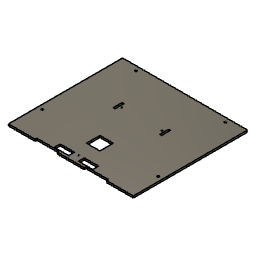
tablet_back_plate (Autodesk Fusion 360 design; units mm, degrees)
Autodesk Fusion 360 part; units mm, degrees
note: some values were not read from the file. Set by a fixed rule: the direction of a hole.
sketch "スケッチ1" plane through (0, 0, 0) normal (0, 1, 0) x (1, 0, 0)
  line L0 (140, 0) -> (140, 256)
  line L1 (140, 256) -> (-140, 256)
  line L2 (-140, 256) -> (-140, 0)
  line L3 (-54, 169) -> (-50, 169)
  line L4 (-50, 169) -> (-50, 149)
  line L5 (-50, 149) -> (-54, 149)
  line L6 (-54, 149) -> (-54, 169)
  line L7 (50, 169) -> (54, 169)
  line L8 (54, 169) -> (54, 149)
  line L9 (54, 149) -> (50, 149)
  line L10 (50, 149) -> (50, 169)
  line L11 (-50, 159) -> (-45, 159)
  line L12 (50, 159) -> (45, 159)
  line L13 (-130, 66) -> (-130, 246)
  line L14 (-130, 246) -> (130, 246)
  line L15 (130, 246) -> (130, 66)
  line L16 (-140, 0) -> (-80, 0)
  line L17 (-80, 0) -> (-80, 4)
  line L18 (-80, 4) -> (-30, 4)
  line L19 (-30, 4) -> (-30, 0)
  line L20 (-30, 0) -> (30, 0)
  line L21 (30, 0) -> (30, 4)
  line L22 (30, 4) -> (80, 4)
  line L23 (80, 4) -> (80, 0)
  line L24 (80, 0) -> (140, 0)
  line L25 (0, 0) -> (0, 17.5)
  line L26 (15, 80) -> (-15, 80)
  line L27 (-15, 80) -> (-15, 50)
  line L28 (-15, 50) -> (15, 50)
  line L29 (15, 50) -> (15, 80)
  line L30 (15, 80) -> (-15, 50) construction
  line L31 (-15, 80) -> (15, 50) construction
  point P0 (-100, 246)
  point P1 (100, 246)
  point P2 (0, 65)
  dimension "d1" = 256
  dimension "d4" = 50
  dimension "d6" = 20
  dimension "d7" = 4
  dimension "d8" = 5
  dimension "d14" = 10
  dimension "d15" = 10
  dimension "d16" = 10
  dimension "d17" = 180
  dimension "d18" = 100
  dimension "d19" = 100
  dimension "d25" = 60
  dimension "d26" = 60
  dimension "d27" = 60
  dimension "d28" = 140
  dimension "d29" = 140
  dimension "d30" = 4
  dimension "d32" = 13.5
  dimension "d33" = 50
  dimension "d34" = 30
  dimension "d35" = 30
  dimension "d41" = 50
  dimension "d42" = 149
  constraint vertical L0
  constraint horizontal L1
  constraint vertical L2
  constraint horizontal L3
  constraint vertical L4
  constraint horizontal L5
  constraint vertical L6
  constraint horizontal L7
  constraint vertical L8
  constraint horizontal L9
  constraint vertical L10
  constraint midpoint L4 L11.start
  constraint perpendicular L4 L11
  constraint midpoint L10 L12.start
  constraint perpendicular L10 L12
  constraint equal L3 L7
  constraint collinear L3 L7
  constraint collinear L5 L9
  constraint equal L11 L12
  constraint vertical L13
  constraint perpendicular L13 L14
  constraint perpendicular L14 L15
  constraint equal L13 L15
  constraint coincident L14 P0
  constraint coincident L14 P1
  constraint perpendicular L2 L16
  constraint perpendicular L16 L17
  constraint perpendicular L17 L18
  constraint perpendicular L16 L19
  constraint perpendicular L19 L20
  constraint perpendicular L20 L21
  constraint perpendicular L19 L22
  constraint perpendicular L22 L23
  constraint perpendicular L23 L24
  constraint coincident L0.start L24
  constraint coincident L0.start L24.end
  constraint collinear L16 L20
  constraint collinear L20 L24
  constraint midpoint L25.start L20
  constraint collinear L18 L22
  constraint coincident L25.start origin
  constraint perpendicular L20 L25
  constraint horizontal L26
  constraint perpendicular L26 L27
  constraint parallel L26 L28
  constraint parallel L27 L29
  constraint coincident L30 P2
  constraint coincident L31 P2
  constraint vertical L25.start P2
  measures "d1" distance of L0.start L0.end
  measures "d4" distance of L25.start L4
  measures "d6" distance of L7.end L8.end
  measures "d7" distance of L8.end L9.end
  measures "d8" distance of L12.start L12.end
  measures "d14" distance of L1 L14
  measures "d15" distance of L2 L13
  measures "d16" distance of L0 L15
  measures "d17" distance of L13.start L13.end
  measures "d18" horizontal distance of L25.start P0
  measures "d19" horizontal distance of L25.start P1
  measures "d25" distance of L19.end L20.end
  measures "d26" distance of L2.end L16.end
  measures "d27" distance of L23.end L0.start
  measures "d28" distance of L25.start L2
  measures "d29" distance of L25.start L0
  measures "d30" distance of L18 L20
  measures "d32" distance of L18 L25.end
  measures "d33" distance of L20 L28
  measures "d34" distance of L26.end L27.end
  measures "d35" distance of L26.start L26.end
  measures "d41" distance of L25.start L10
  measures "d42" distance of L25.start L9
extrude "押し出し1" add sketch "スケッチ1" along normal blind 4
hole "穴1" at (-45, 0, -159) at (45, 0, -159) at (0, 0, -17.5) direction (0, 1, 0) diameter 3.2 depth 4 tip angle 118
hole "穴2" at (100, 0, -246) at (130, 0, -66) at (-130, 0, -66) at (-100, 0, -246) direction (0, 1, 0) diameter 4.3 end through all
fillet "フィレット1" radius 1 2 edges at (140, 2, -256) (-140, 2, -256)
sketch "スケッチ2" plane through (0, 4, 0) normal (0, 1, 0) x (-1, 0, 0)
  arc A0 (139, -256) -> (140, -255) centre (139, -255) ccw
  line L0 (140, -255) -> (140, 0)
  line L1 (140, 0) -> (80, 0)
  line L2 (80, 0) -> (80, -4)
  line L3 (80, -4) -> (30, -4)
  line L4 (30, -4) -> (30, 0)
  line L5 (30, 0) -> (-30, 0)
  line L6 (-30, 0) -> (-30, -4)
  line L7 (-30, -4) -> (-80, -4)
  line L8 (-80, -4) -> (-80, 0)
  line L9 (-80, 0) -> (-140, 0)
  line L10 (-140, 0) -> (-140, -255)
  arc A1 (-140, -255) -> (-139, -256) centre (-139, -255) ccw
  line L11 (-139, -256) -> (139, -256)
  circle A2 centre (130, -66) radius 2.15
  circle A3 centre (-100, -246) radius 2.15
  circle A4 centre (-130, -66) radius 2.15
  circle A5 centre (100, -246) radius 2.15
  circle A6 centre (-45, -159) radius 1.6
  circle A7 centre (45, -159) radius 1.6
  circle A8 centre (0, -17.5) radius 1.6
  line L12 (-54, -149) -> (-50, -149)
  line L13 (-50, -149) -> (-50, -169)
  line L14 (-50, -169) -> (-54, -169)
  line L15 (-54, -169) -> (-54, -149)
  line L16 (-15, -80) -> (-15, -50)
  line L17 (-15, -50) -> (15, -50)
  line L18 (15, -50) -> (15, -80)
  line L19 (15, -80) -> (-15, -80)
  line L20 (50, -149) -> (54, -149)
  line L21 (54, -149) -> (54, -169)
  line L22 (54, -169) -> (50, -169)
  line L23 (50, -169) -> (50, -149)
  line L24 (-43, -6) -> (-11, -6)
  line L25 (-11, -6) -> (-11, -19)
  line L26 (-11, -19) -> (-43, -19)
  line L27 (-43, -19) -> (-43, -6)
  line L28 (43, -19) -> (11, -19)
  line L29 (11, -19) -> (11, -6)
  line L30 (11, -6) -> (43, -6)
  line L31 (43, -6) -> (43, -19)
  dimension "d43" = 6
  dimension "d44" = 11
  dimension "d45" = 32
  dimension "d46" = 13
  dimension "d47" = 11
  dimension "d48" = 32
  constraint horizontal L24
  constraint vertical L25
  constraint horizontal L26
  constraint vertical L27
  constraint horizontal L28
  constraint vertical L29
  constraint horizontal L30
  constraint vertical L31
  constraint collinear L26 L28
  constraint collinear L24 L30
  measures "d43" distance of L5 L24
  measures "d44" distance of origin L25
  measures "d45" distance of L25.end L26.end
  measures "d46" distance of L24.start L26.end
  measures "d47" distance of origin L29
  measures "d48" distance of L28.start L28.end
extrude "押し出し2" cut sketch "スケッチ2" against normal through all contours L24 L25 L26 L27 | L28 L29 L30 L31
